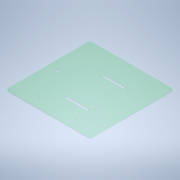
# Autodesk Inventor part: Old case New Board Adapter
Saved by Autodesk Inventor 2022 (Build 260153000, 153)
## iProperties
Created: 2021-06-16
Part Number: Old case New Board Adapter
Material: Glass
Document SubType Name: Modeling
Designer: benka
Density: 2.18 g/cm^3
Appearance: Clear - Green 1
Author: benka
Autodesk Inventor part; units mm, degrees
ref_plane "YZ Plane" through (0, 0, 0) normal (1, 0, 0) x (0, 1, 0)
ref_plane "XZ Plane" through (0, 0, 0) normal (0, 1, 0) x (-1, 0, 0)
ref_plane "XY Plane" through (0, 0, 0) normal (0, 0, 1) x (1, 0, 0)
sketch "Sketch1" plane through (0, 0, 0) normal (0, 1, 0) x (-1, 0, 0)
  line L0 (-90, 95) -> (90, 95)
  line L1 (95, 90) -> (95, -90)
  line L2 (90, -95) -> (-90, -95)
  line L3 (-95, -90) -> (-95, 90)
  line L4 (-37.5033, 38.736) -> (-37.5033, 44.686)
  line L5 (-37.5033, 44.686) -> (14.5465, 44.686)
  line L6 (14.5465, 44.686) -> (14.5465, 38.736)
  line L7 (14.5465, 38.736) -> (-37.5033, 38.736)
  line L8 (-37.4788, -45.2638) -> (-37.4788, -39.3138)
  line L9 (-37.4788, -39.3138) -> (14.5465, -39.3138)
  line L10 (14.5465, -39.3138) -> (14.5465, -45.2638)
  line L11 (14.5465, -45.2638) -> (-37.4788, -45.2638)
  circle A0 centre (41.7215, 73.186) radius 1.2478
  circle A1 centre (73.2215, -0.3141) radius 3.7486
  circle A2 centre (41.7215, -73.8137) radius 1.2732
  circle A3 centre (-42.2782, -73.8137) radius 1.2727
  circle A4 centre (-42.2783, 73.186) radius 1.2728
  circle A5 centre (89.6714, 89.8399) radius 1.5
  circle A6 centre (89.671, -90.1601) radius 1.5
  circle A7 centre (-90.329, -90.1601) radius 1.5
  circle A8 centre (-90.3286, 89.8399) radius 1.5
  arc A9 (90, -95) -> (95, -90) centre (90, -90) ccw
  arc A10 (-95, -90) -> (-90, -95) centre (-90, -90) ccw
  arc A11 (-90, 95) -> (-95, 90) centre (-90, 90) ccw
  arc A12 (95, 90) -> (90, 95) centre (90, 90) ccw
  point P0 (-95, 95)
  point P1 (95, 95)
  point P2 (95, -95)
  point P3 (-95, -95)
  point P4 (0, 0)
  point P5 (0, 0)
  dimension "d4" = 3
  dimension "d0" = 3
  dimension "d1" = 3
  dimension "d2" = 3
  dimension "d3" = 3
  dimension "d6" = 5
  dimension "d7" = 95
  dimension "d8" = 95
  dimension "d9" = 180
  dimension "d10" = 180
  dimension "d11" = 180
  dimension "d12" = 180
  dimension "d13" = 190
  dimension "d14" = 190
  dimension "d15" = 73.5001
  dimension "d16" = 31.5
  dimension "d17" = 95
  dimension "d18" = 95
  constraints: 24 end point, 13 centre point, 8 point on circle, 8 point on line, 8 tangent, 3 equal radius
  measures "d0" diameter of A5
  measures "d1" diameter of A6
  measures "d2" diameter of A7
  measures "d3" diameter of A8
  measures "d6" radius of A9
  measures "d7" distance from line of L0 point (0, 0)
  measures "d8" distance from line of L2 point (0, 0)
  measures "d9" distance of A7.centre A6.centre
  measures "d10" distance of A5.centre A6.centre
  measures "d11" distance of A8.centre A7.centre
  measures "d12" distance of A5.centre A8.centre
  measures "d13" distance between parallel lines of L3 L1
  measures "d14" distance between parallel lines of L0 L2
  measures "d15" vertical distance of A0.centre A1.centre
  measures "d16" horizontal distance of A1.centre A0.centre
  measures "d17" distance from line of L3 point (0, 0)
  measures "d18" distance from line of point (0, 0) L1
extrude "Extrusion1" add sketch "Sketch1" along normal blind 3
body "Solid1"
